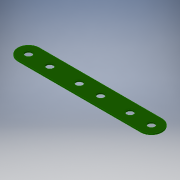
# Autodesk Inventor part: TubePCB
Saved by Autodesk Inventor 2017 (Build 210142000, 142)
## iProperties
Created: 2017-04-16
Part Number: TubePCB
Material: Generic
Document SubType Name: Modeling
Designer: jeffkub
Density: 1 g/cm^3
Appearance: Default(3)
Author: jeffkub
Autodesk Inventor part; units mm, degrees
ref_plane "YZ Plane" through (0, 0, 0) normal (1, 0, 0) x (0, 1, 0)
ref_plane "XZ Plane" through (0, 0, 0) normal (0, 1, 0) x (-1, 0, 0)
ref_plane "XY Plane" through (0, 0, 0) normal (0, 0, 1) x (1, 0, 0)
sketch "Sketch1" plane through (0, 0, 0) normal (0, 1, 0) x (-1, 0, 0)
  line L0 (-75, 0) -> (75, 0) construction
  line L1 (-75, -13) -> (75, -13)
  line L2 (75, 13) -> (-75, 13)
  arc A0 (-75, 13) -> (-75, -13) centre (-75, 0) ccw
  arc A1 (75, -13) -> (75, 13) centre (75, 0) ccw
  circle A2 centre (75, 0) radius 4.3
  circle A3 centre (49, 0) radius 4.3
  circle A4 centre (13, 0) radius 4.3
  circle A5 centre (-13, 0) radius 4.3
  circle A6 centre (-49, 0) radius 4.3
  circle A7 centre (-75, 0) radius 4.3
  point P0 (0, 0)
  dimension "d0" = 150
  dimension "d1" = 26
  dimension "d2" = 8.6
  dimension "d3" = 26
  dimension "d6" = 62
  constraints: 8 centre point, 8 end point, 4 point on circle, 4 tangent, 2 horizontal, 1 coincident, 1 equal radius, 1 midpoint, 1 parallel, 1 point on line, 8 other
  measures "d0" distance of L0.start L0.end
  measures "d1" distance between parallel lines of L2 L1
  measures "d2" diameter of A2
  measures "d3" distance of A3.centre L0.end
  measures "d6" distance of A2.centre A4.centre
extrude "Extrusion1" add sketch "Sketch1" along normal blind 1.6
body "Solid1"
